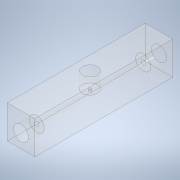
# Autodesk Inventor part: T-Sensor_PT100
Saved by Autodesk Inventor 2022 (Build 260153000, 153)
## iProperties
Created: 2021-06-08
Part Number: T-Sensor_PT100
Material: PMMA-Kunststoff
Document SubType Name: Modeling
Designer: smlehelw
Density: 1.188 g/cm^3
Appearance: Polycarbonat - klar
Author: smlehelw
Autodesk Inventor part; units mm, degrees
ref_plane "YZ Plane" through (0, 0, 0) normal (1, 0, 0) x (0, 1, 0)
ref_plane "XZ Plane" through (0, 0, 0) normal (0, 1, 0) x (-1, 0, 0)
ref_plane "XY Plane" through (0, 0, 0) normal (0, 0, 1) x (1, 0, 0)
sketch "Skizze1" plane through (0, 0, 0) normal (0, 1, 0) x (-1, 0, 0)
  line L0 (-5, -25) -> (5, -25)
  line L1 (5, -25) -> (5, 25)
  line L2 (5, 25) -> (-5, 25)
  line L3 (-5, 25) -> (-5, -25)
  line L4 (-5, -25) -> (5, 25) construction
  line L5 (5, -25) -> (-5, 25) construction
  point P0 (0, 0)
  dimension "d0" = 10
  dimension "d1" = 50
  constraints: 12 end point, 2 midpoint, 2 parallel, 1 horizontal, 1 perpendicular
  measures "d0" distance of L2.end L1.end
  measures "d1" distance of L1.end L0.end
extrude "Extrusion1" add sketch "Skizze1" along normal blind 10
sketch "Skizze2" plane through (-5, 0, 25) normal (0, 0, 1) x (1, 0, 0)
  circle A0 centre (5, 5) radius 0.8
  point P0 (5, 0)
  dimension "d4" = 1.6
  constraints: 1 centre point
  measures "d4" diameter of A0
hole "Bohrung1" at (0, 5, 25) direction (0, 0, -1) diameter 1.6 end through all
sketch "Skizze3" plane through (0, 10, 0) normal (0, 1, 0) x (1, 0, 0)
  point P0 (0, 0)
sketch "Skizze4" plane through (0, 10, 0) normal (0, 1, 0) x (1, 0, 0)
  point P0 (0, 0)
sketch "Skizze5" plane through (0, 10, 0) normal (0, 1, 0) x (1, 0, 0)
  line L0 (-5, 25) -> (-5, -25) projected
  line L1 (5, -25) -> (5, 25) projected
  line L2 (-5, -25) -> (5, -25)
  line L3 (5, -25) -> (5, 25)
  line L4 (5, 25) -> (-5, 25)
  line L5 (-5, 25) -> (-5, -25)
  point P0 (0, 0)
  constraints: 8 end point, 2 parallel, 1 horizontal, 1 perpendicular
extrude "Extrusion2" add sketch "Skizze5" along normal blind 2
sketch "Skizze6" plane through (0, 12, 0) normal (0, 1, 0) x (1, 0, 0)
  point P0 (0, 0)
hole "Bohrung2" at (0, 12, 0) direction (0, -1, 0) diameter 1 depth 6.7
sketch "Skizze7" plane through (0, 12, 0) normal (0, 1, 0) x (1, 0, 0)
  point P0 (0, 0)
hole "Bohrung3" at (0, 12, 0) direction (0, -1, 0) diameter 5.4 depth 5.7
sketch "Skizze8" plane through (-5, 0, 25) normal (0, 0, 1) x (1, 0, 0)
  circle A0 centre (5, 5.0108) radius 1.4918
  point P0 (5, 0)
  constraints: 1 centre point
hole "Bohrung4" at (0, 5.0108, 25) direction (0, 0, -1) diameter 5.4 depth 5.7
sketch "Skizze9" plane through (5, 0, -25) normal (0, 0, -1) x (-1, 0, 0)
  circle A0 centre (5, 5) radius 0.8 projected
  circle A1 centre (5, 5) radius 2.7
  point P0 (5, 0)
  dimension "d35" = 5.4
  constraints: 1 centre point, 1 coincident
  measures "d35" diameter of A1
hole "Bohrung5" at (0, 5, -25) direction (0, 0, 1) diameter 5.4 depth 5.7
